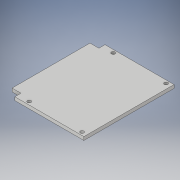
# Autodesk Inventor part: 000,105 - Дно переднего сегмента
Saved by Autodesk Inventor 2019 (Build 230136000, 136)
## iProperties
Created: 2020-06-06
Part Number: 000,105 - Дно переднего сегмента
Material: Типовые
Document SubType Name: Modeling
Designer: Петров Иван
Density: 1 g/cm^3
Appearance: По умолчанию
Author: Петров Иван
Autodesk Inventor part; units mm, degrees
ref_plane "YZ Plane" through (0, 0, 0) normal (1, 0, 0) x (0, 1, 0)
ref_plane "XZ Plane" through (0, 0, 0) normal (0, 1, 0) x (-1, 0, 0)
ref_plane "XY Plane" through (0, 0, 0) normal (0, 0, 1) x (1, 0, 0)
sketch "Эскиз1" plane through (0, 0, 0) normal (0, 1, 0) x (-1, 0, 0)
  circle A0 centre (51.875, 2.75) radius 1.6
  circle A1 centre (4.375, 2.75) radius 1.6
  line L0 (0, 5.5) -> (62, 5.5)
  line L1 (0, 0) -> (0, 5.5)
  line L2 (62, 0) -> (0, 0)
  line L3 (62, 5.5) -> (62, 0)
  circle A2 centre (51.875, -72.75) radius 1.6
  circle A3 centre (4.375, -72.75) radius 1.6
  line L4 (0, -75.5) -> (62, -75.5)
  line L5 (62, -75.5) -> (62, -70)
  line L6 (0, -70) -> (62, -70)
  line L7 (0, -70) -> (0, -75.5)
  line L8 (70, -70) -> (62, -70)
  line L9 (70, -70) -> (70, -55)
  line L10 (70, -55) -> (70, -15)
  line L11 (70, -15) -> (70, 0)
  line L12 (70, 0) -> (62, 0)
  line L13 (0, -15) -> (0, -55)
  line L14 (0, 0) -> (0, -15)
  line L15 (0, -55) -> (0, -70)
  point P0 (35, -35)
  constraints: 32 end point, 4 centre point
extrude "Выдавливание1" add sketch "Эскиз1" along normal blind 3
